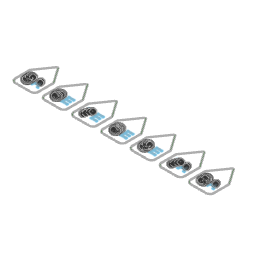
6-9 (Autodesk Fusion 360 design; units mm, degrees)
Autodesk Fusion 360 part; units mm, degrees
(part 1 of 2)
sketch "Sketch1" plane through (0, 0, 1) normal (0, 0, 1) x (-1, 0, 0)
  arc A0 (14.0709, -45.9158) -> (17.3475, -45.9158) centre (15.7092, -44.7687) ccw
  line L0 (17.3475, -45.9158) -> (31.3664, -25.8947)
  arc A1 (31.3664, -25.8947) -> (31.7281, -24.7475) centre (29.7281, -24.7475) ccw
  line L1 (31.7281, -24.7475) -> (31.7281, -6.3281)
  arc A2 (31.7281, -6.3281) -> (25.4, 0) centre (25.4, -6.3281) ccw
  line L2 (25.4, 0) -> (6.0183, 0)
  arc A3 (6.0183, 0) -> (0, -4.3724) centre (6.0183, -6.3281) ccw
  line L3 (0, -4.3724) -> (0, -25.19)
  arc A4 (0, -25.19) -> (0.3617, -26.3371) centre (2, -25.19) ccw
  line L4 (0.3617, -26.3371) -> (14.0709, -45.9158)
  arc A5 (-24.0291, -45.9158) -> (-20.7525, -45.9158) centre (-22.3908, -44.7687) ccw
  line L5 (-20.7525, -45.9158) -> (-6.7336, -25.8947)
  arc A6 (-6.7336, -25.8947) -> (-6.3719, -24.7475) centre (-8.3719, -24.7475) ccw
  line L6 (-6.3719, -24.7475) -> (-6.3719, -6.3281)
  arc A7 (-6.3719, -6.3281) -> (-12.7, 0) centre (-12.7, -6.3281) ccw
  line L7 (-12.7, 0) -> (-32.0817, 0)
  arc A8 (-32.0817, 0) -> (-38.1, -4.3724) centre (-32.0817, -6.3281) ccw
  line L8 (-38.1, -4.3724) -> (-38.1, -25.19)
  arc A9 (-38.1, -25.19) -> (-37.7383, -26.3371) centre (-36.1, -25.19) ccw
  line L9 (-37.7383, -26.3371) -> (-24.0291, -45.9158)
  arc A10 (-62.1291, -45.9158) -> (-58.8525, -45.9158) centre (-60.4908, -44.7687) ccw
  line L10 (-58.8525, -45.9158) -> (-44.8336, -25.8947)
  arc A11 (-44.8336, -25.8947) -> (-44.4719, -24.7475) centre (-46.4719, -24.7475) ccw
  line L11 (-44.4719, -24.7475) -> (-44.4719, -6.3281)
  arc A12 (-44.4719, -6.3281) -> (-50.8, 0) centre (-50.8, -6.3281) ccw
  line L12 (-50.8, 0) -> (-70.1817, 0)
  arc A13 (-70.1817, 0) -> (-76.2, -4.3724) centre (-70.1817, -6.3281) ccw
  line L13 (-76.2, -4.3724) -> (-76.2, -25.19)
  arc A14 (-76.2, -25.19) -> (-75.8383, -26.3371) centre (-74.2, -25.19) ccw
  line L14 (-75.8383, -26.3371) -> (-62.1291, -45.9158)
  arc A15 (-100.2291, -45.9158) -> (-96.9525, -45.9158) centre (-98.5908, -44.7687) ccw
  line L15 (-96.9525, -45.9158) -> (-82.9336, -25.8947)
  arc A16 (-82.9336, -25.8947) -> (-82.5719, -24.7475) centre (-84.5719, -24.7475) ccw
  line L16 (-82.5719, -24.7475) -> (-82.5719, -6.3281)
  arc A17 (-82.5719, -6.3281) -> (-88.9, 0) centre (-88.9, -6.3281) ccw
  line L17 (-88.9, 0) -> (-108.2817, 0)
  arc A18 (-108.2817, 0) -> (-114.3, -4.3724) centre (-108.2817, -6.3281) ccw
  line L18 (-114.3, -4.3724) -> (-114.3, -25.19)
  arc A19 (-114.3, -25.19) -> (-113.9383, -26.3371) centre (-112.3, -25.19) ccw
  line L19 (-113.9383, -26.3371) -> (-100.2291, -45.9158)
  arc A20 (-138.3291, -45.9158) -> (-135.0525, -45.9158) centre (-136.6908, -44.7687) ccw
  line L20 (-135.0525, -45.9158) -> (-121.0336, -25.8947)
  arc A21 (-121.0336, -25.8947) -> (-120.6719, -24.7475) centre (-122.6719, -24.7475) ccw
  line L21 (-120.6719, -24.7475) -> (-120.6719, -6.3281)
  arc A22 (-120.6719, -6.3281) -> (-127, 0) centre (-127, -6.3281) ccw
  line L22 (-127, 0) -> (-146.3817, 0)
  arc A23 (-146.3817, 0) -> (-152.4, -4.3724) centre (-146.3817, -6.3281) ccw
  line L23 (-152.4, -4.3724) -> (-152.4, -25.19)
  arc A24 (-152.4, -25.19) -> (-152.0383, -26.3371) centre (-150.4, -25.19) ccw
  line L24 (-152.0383, -26.3371) -> (-138.3291, -45.9158)
  arc A25 (-176.4291, -45.9158) -> (-173.1525, -45.9158) centre (-174.7908, -44.7687) ccw
  line L25 (-173.1525, -45.9158) -> (-159.1336, -25.8947)
  arc A26 (-159.1336, -25.8947) -> (-158.7719, -24.7475) centre (-160.7719, -24.7475) ccw
  line L26 (-158.7719, -24.7475) -> (-158.7719, -6.3281)
  arc A27 (-158.7719, -6.3281) -> (-165.1, 0) centre (-165.1, -6.3281) ccw
  line L27 (-165.1, 0) -> (-184.4817, 0)
  arc A28 (-184.4817, 0) -> (-190.5, -4.3724) centre (-184.4817, -6.3281) ccw
  line L28 (-190.5, -4.3724) -> (-190.5, -25.19)
  arc A29 (-190.5, -25.19) -> (-190.1383, -26.3371) centre (-188.5, -25.19) ccw
  line L29 (-190.1383, -26.3371) -> (-176.4291, -45.9158)
  arc A30 (-214.5291, -45.9158) -> (-211.2525, -45.9158) centre (-212.8908, -44.7687) ccw
  line L30 (-211.2525, -45.9158) -> (-197.2336, -25.8947)
  arc A31 (-197.2336, -25.8947) -> (-196.8719, -24.7475) centre (-198.8719, -24.7475) ccw
  line L31 (-196.8719, -24.7475) -> (-196.8719, -6.3281)
  arc A32 (-196.8719, -6.3281) -> (-203.2, 0) centre (-203.2, -6.3281) ccw
  line L32 (-203.2, 0) -> (-222.5817, 0)
  arc A33 (-222.5817, 0) -> (-228.6, -4.3724) centre (-222.5817, -6.3281) ccw
  line L33 (-228.6, -4.3724) -> (-228.6, -25.19)
  arc A34 (-228.6, -25.19) -> (-228.2383, -26.3371) centre (-226.6, -25.19) ccw
  line L34 (-228.2383, -26.3371) -> (-214.5291, -45.9158)
  line L35 (16.1187, -45.0555) -> (30.1377, -25.0343)
  arc A35 (30.1377, -25.0343) -> (30.2281, -24.7475) centre (29.7281, -24.7475) ccw
  line L36 (30.2281, -24.7475) -> (30.2281, -6.3281)
  arc A36 (30.2281, -6.3281) -> (25.4, -1.5) centre (25.4, -6.3281) ccw
  line L37 (25.4, -1.5) -> (6.0183, -1.5)
  arc A37 (6.0183, -1.5) -> (1.5, -4.6265) centre (6.0183, -6.3281) ccw
  line L38 (1.5, -4.6265) -> (1.5, -25.19)
  arc A38 (1.5, -25.19) -> (1.5904, -25.4768) centre (2, -25.19) ccw
  line L39 (1.5904, -25.4768) -> (15.2996, -45.0555)
  arc A39 (15.2996, -45.0555) -> (16.1187, -45.0555) centre (15.7092, -44.7687) ccw
  line L40 (-21.9813, -45.0555) -> (-7.9623, -25.0343)
  arc A40 (-7.9623, -25.0343) -> (-7.8719, -24.7475) centre (-8.3719, -24.7475) ccw
  line L41 (-7.8719, -24.7475) -> (-7.8719, -6.3281)
  arc A41 (-7.8719, -6.3281) -> (-12.7, -1.5) centre (-12.7, -6.3281) ccw
  line L42 (-12.7, -1.5) -> (-32.0817, -1.5)
  arc A42 (-32.0817, -1.5) -> (-36.6, -4.6265) centre (-32.0817, -6.3281) ccw
  line L43 (-36.6, -4.6265) -> (-36.6, -25.19)
  arc A43 (-36.6, -25.19) -> (-36.5096, -25.4768) centre (-36.1, -25.19) ccw
  line L44 (-36.5096, -25.4768) -> (-22.8004, -45.0555)
  arc A44 (-22.8004, -45.0555) -> (-21.9813, -45.0555) centre (-22.3908, -44.7687) ccw
  line L45 (-60.0813, -45.0555) -> (-46.0623, -25.0343)
  arc A45 (-46.0623, -25.0343) -> (-45.9719, -24.7475) centre (-46.4719, -24.7475) ccw
  line L46 (-45.9719, -24.7475) -> (-45.9719, -6.3281)
  arc A46 (-45.9719, -6.3281) -> (-50.8, -1.5) centre (-50.8, -6.3281) ccw
  line L47 (-50.8, -1.5) -> (-70.1817, -1.5)
  arc A47 (-70.1817, -1.5) -> (-74.7, -4.6265) centre (-70.1817, -6.3281) ccw
  line L48 (-74.7, -4.6265) -> (-74.7, -25.19)
  arc A48 (-74.7, -25.19) -> (-74.6096, -25.4768) centre (-74.2, -25.19) ccw
  line L49 (-74.6096, -25.4768) -> (-60.9004, -45.0555)
  arc A49 (-60.9004, -45.0555) -> (-60.0813, -45.0555) centre (-60.4908, -44.7687) ccw
  line L50 (-98.1813, -45.0555) -> (-84.1623, -25.0343)
  arc A50 (-84.1623, -25.0343) -> (-84.0719, -24.7475) centre (-84.5719, -24.7475) ccw
  line L51 (-84.0719, -24.7475) -> (-84.0719, -6.3281)
  arc A51 (-84.0719, -6.3281) -> (-88.9, -1.5) centre (-88.9, -6.3281) ccw
  line L52 (-88.9, -1.5) -> (-108.2817, -1.5)
  arc A52 (-108.2817, -1.5) -> (-112.8, -4.6265) centre (-108.2817, -6.3281) ccw
  line L53 (-112.8, -4.6265) -> (-112.8, -25.19)
  arc A53 (-112.8, -25.19) -> (-112.7096, -25.4768) centre (-112.3, -25.19) ccw
  line L54 (-112.7096, -25.4768) -> (-99.0004, -45.0555)
  arc A54 (-99.0004, -45.0555) -> (-98.1813, -45.0555) centre (-98.5908, -44.7687) ccw
  line L55 (-136.2813, -45.0555) -> (-122.2623, -25.0343)
  arc A55 (-122.2623, -25.0343) -> (-122.1719, -24.7475) centre (-122.6719, -24.7475) ccw
  line L56 (-122.1719, -24.7475) -> (-122.1719, -6.3281)
  arc A56 (-122.1719, -6.3281) -> (-127, -1.5) centre (-127, -6.3281) ccw
  line L57 (-127, -1.5) -> (-146.3817, -1.5)
  arc A57 (-146.3817, -1.5) -> (-150.9, -4.6265) centre (-146.3817, -6.3281) ccw
  line L58 (-150.9, -4.6265) -> (-150.9, -25.19)
  arc A58 (-150.9, -25.19) -> (-150.8096, -25.4768) centre (-150.4, -25.19) ccw
  line L59 (-150.8096, -25.4768) -> (-137.1004, -45.0555)
  arc A59 (-137.1004, -45.0555) -> (-136.2813, -45.0555) centre (-136.6908, -44.7687) ccw
  line L60 (-160.2719, -24.7475) -> (-160.2719, -6.3281)
  arc A60 (-160.2719, -6.3281) -> (-165.1, -1.5) centre (-165.1, -6.3281) ccw
  line L61 (-165.1, -1.5) -> (-184.4817, -1.5)
  arc A61 (-184.4817, -1.5) -> (-189, -4.6265) centre (-184.4817, -6.3281) ccw
  line L62 (-189, -4.6265) -> (-189, -25.19)
  arc A62 (-189, -25.19) -> (-188.9096, -25.4768) centre (-188.5, -25.19) ccw
  line L63 (-188.9096, -25.4768) -> (-175.2004, -45.0555)
  arc A63 (-175.2004, -45.0555) -> (-174.3813, -45.0555) centre (-174.7908, -44.7687) ccw
  line L64 (-174.3813, -45.0555) -> (-160.3623, -25.0343)
  arc A64 (-160.3623, -25.0343) -> (-160.2719, -24.7475) centre (-160.7719, -24.7475) ccw
  line L65 (-212.4813, -45.0555) -> (-198.4623, -25.0343)
  arc A65 (-198.4623, -25.0343) -> (-198.3719, -24.7475) centre (-198.8719, -24.7475) ccw
  line L66 (-198.3719, -24.7475) -> (-198.3719, -6.3281)
  arc A66 (-198.3719, -6.3281) -> (-203.2, -1.5) centre (-203.2, -6.3281) ccw
  line L67 (-203.2, -1.5) -> (-222.5817, -1.5)
  arc A67 (-222.5817, -1.5) -> (-227.1, -4.6265) centre (-222.5817, -6.3281) ccw
  line L68 (-227.1, -4.6265) -> (-227.1, -25.19)
  arc A68 (-227.1, -25.19) -> (-227.0096, -25.4768) centre (-226.6, -25.19) ccw
  line L69 (-227.0096, -25.4768) -> (-213.3004, -45.0555)
  arc A69 (-213.3004, -45.0555) -> (-212.4813, -45.0555) centre (-212.8908, -44.7687) ccw
  line L70 (-7.9796, -5.9789) -> (-36.2077, -5.9789) construction
  line L71 (-36.2077, -5.9789) -> (-36.2077, -24.6143) construction
  line L72 (-36.2077, -24.6143) -> (-7.9796, -24.6143) construction
  line L73 (-7.9796, -24.6143) -> (-7.9796, -5.9789) construction
  line L74 (-46.2203, -6.1121) -> (-74.4484, -6.1121) construction
  line L75 (-74.4484, -6.1121) -> (-74.4484, -24.7475) construction
  line L76 (-74.4484, -24.7475) -> (-46.2203, -24.7475) construction
  line L77 (-46.2203, -24.7475) -> (-46.2203, -6.1121) construction
  line L78 (-84.8121, -6.1121) -> (-113.0403, -6.1121) construction
  line L79 (-113.0403, -6.1121) -> (-113.0403, -24.7475) construction
  line L80 (-113.0403, -24.7475) -> (-84.8121, -24.7475) construction
  line L81 (-84.8121, -24.7475) -> (-84.8121, -6.1121) construction
  line L82 (29.7281, -6.1121) -> (1.5, -6.1121) construction
  line L83 (1.5, -6.1121) -> (1.5, -24.7475) construction
  line L84 (1.5, -24.7475) -> (29.7281, -24.7475) construction
  line L85 (29.7281, -24.7475) -> (29.7281, -6.1121) construction
  line L86 (-122.5602, -5.9501) -> (-150.7883, -5.9501) construction
  line L87 (-150.7883, -5.9501) -> (-150.7883, -24.5855) construction
  line L88 (-150.7883, -24.5855) -> (-122.5602, -24.5855) construction
  line L89 (-122.5602, -24.5855) -> (-122.5602, -5.9501) construction
  line L90 (-160.6323, -6.4361) -> (-188.8604, -6.4361) construction
  line L91 (-188.8604, -6.4361) -> (-188.8604, -25.0715) construction
  line L92 (-188.8604, -25.0715) -> (-160.6323, -25.0715) construction
  line L93 (-160.6323, -25.0715) -> (-160.6323, -6.4361) construction
  line L94 (-199.0284, -6.1121) -> (-227.2565, -6.1121) construction
  line L95 (-227.2565, -6.1121) -> (-227.2565, -24.7475) construction
  line L96 (-227.2565, -24.7475) -> (-199.0284, -24.7475) construction
  line L97 (-199.0284, -24.7475) -> (-199.0284, -6.1121) construction
  dimension "d1" = -1.5
  dimension "d2" = -1.5
  dimension "d3" = -1.5
  dimension "d4" = -1.5
  dimension "d5" = -1.5
  dimension "d6" = -1.5
  dimension "d7" = -1.5
sketch "sketch 2408" plane through (0, 0, 1) normal (0, 0, 1) x (-1, 0, 0)
  line L0 (11.1666, -17.4709) -> (12.2657, -14.5356)
  spline S0 degree 3 poles (10.6273, -19.3824) (10.698, -19.0609) (10.8404, -18.4133) (11.0574, -17.7866) (11.1666, -17.4709) knots 0 0 0 0 0.09864 0.198754 0.198754 0.198754 0.198754
  spline S1 degree 3 poles (9.9174, -17.3071) (10.0605, -17.6891) (10.3171, -18.374) (10.5322, -19.0731) (10.6273, -19.3824) knots 0 0 0 0 0.122331 0.219376 0.219376 0.219376 0.219376
  line L1 (8.8729, -14.5356) -> (9.9174, -17.3071)
  line L2 (12.2657, -14.5356) -> (8.8729, -14.5356)
  line L3 (13.747, -10.426) -> (15.1533, -10.426)
  line L4 (12.648, -13.457) -> (13.747, -10.426)
  line L5 (8.4633, -13.457) -> (12.648, -13.457)
  line L6 (7.296, -10.426) -> (8.4633, -13.457)
  line L7 (5.7874, -10.426) -> (7.296, -10.426)
  line L8 (9.8832, -20.4336) -> (5.7874, -10.426)
  line L9 (11.31, -20.4336) -> (9.8832, -20.4336)
  line L10 (15.1533, -10.426) -> (11.31, -20.4336)
  spline S2 degree 3 poles (24.3622, -10.9073) (24.5865, -11.1558) (25.0592, -11.6795) (25.1885, -12.3748) (25.2564, -12.7402) knots 0 0 0 0 0.098474 0.207515 0.207515 0.207515 0.207515
  spline S3 degree 3 poles (22.4439, -10.2554) (22.8109, -10.277) (23.5118, -10.3184) (24.0878, -10.7173) (24.3622, -10.9073) knots 0 0 0 0 0.107902 0.2061 0.2061 0.2061 0.2061
  spline S4 degree 3 poles (20.5155, -10.8493) (20.8056, -10.6761) (21.3995, -10.3215) (22.0905, -10.2777) (22.4439, -10.2554) knots 0 0 0 0 0.099829 0.204395 0.204395 0.204395 0.204395
  spline S5 degree 3 poles (19.2765, -12.5798) (19.4252, -12.2287) (19.7093, -11.5582) (20.2553, -11.0781) (20.5155, -10.8493) knots 0 0 0 0 0.112701 0.215277 0.215277 0.215277 0.215277
  spline S6 degree 3 poles (18.86, -15.6346) (18.8678, -15.0564) (18.8817, -14.0198) (19.1554, -13.0213) (19.2765, -12.5798) knots 0 0 0 0 0.172597 0.309411 0.309411 0.309411 0.309411
  spline S7 degree 3 poles (19.2799, -18.4505) (19.158, -18.0565) (18.875, -17.1412) (18.8655, -16.1813) (18.86, -15.6346) knots 0 0 0 0 0.123131 0.286024 0.286024 0.286024 0.286024
  spline S8 degree 3 poles (20.5086, -19.9489) (20.2536, -19.7512) (19.7303, -19.3457) (19.4325, -18.7538) (19.2799, -18.4505) knots 0 0 0 0 0.095539 0.195973 0.195973 0.195973 0.195973
  spline S9 degree 3 poles (22.2938, -20.4746) (21.9758, -20.453) (21.3418, -20.4098) (20.7858, -20.1023) (20.5086, -19.9489) knots 0 0 0 0 0.094357 0.188122 0.188122 0.188122 0.188122
  spline S10 degree 3 poles (24.5431, -19.5462) (24.2221, -19.817) (23.5718, -20.3656) (22.7234, -20.4379) (22.2938, -20.4746) knots 0 0 0 0 0.122772 0.248744 0.248744 0.248744 0.248744
  spline S11 degree 3 poles (25.4408, -17.0955) (25.4107, -17.5703) (25.3532, -18.4783) (24.8048, -19.2013) (24.5431, -19.5462) knots 0 0 0 0 0.139204 0.266205 0.266205 0.266205 0.266205
  spline S12 degree 3 poles (24.5806, -14.7199) (24.8313, -15.0547) (25.3575, -15.7574) (25.4121, -16.6357) (25.4408, -17.0955) knots 0 0 0 0 0.122761 0.257603 0.257603 0.257603 0.257603
  spline S13 degree 3 poles (22.4781, -13.8188) (22.8764, -13.8564) (23.6736, -13.9318) (24.2781, -14.4571) (24.5806, -14.7199) knots 0 0 0 0 0.116876 0.233928 0.233928 0.233928 0.233928
  spline S14 degree 3 poles (21.0957, -14.184) (21.3133, -14.0775) (21.7497, -13.8638) (22.2348, -13.8338) (22.4781, -13.8188) knots 0 0 0 0 0.071895 0.144237 0.144237 0.144237 0.144237
  spline S15 degree 3 poles (20.0888, -15.1363) (20.2245, -14.9489) (20.5002, -14.5683) (20.8952, -14.3134) (21.0957, -14.184) knots 0 0 0 0 0.068756 0.139669 0.139669 0.139669 0.139669
  spline S16 degree 3 poles (20.082, -14.8905) (20.0824, -14.9247) (20.0835, -15.0066) (20.0868, -15.0885) (20.0888, -15.1363) knots 0 0 0 0 0.010241 0.024586 0.024586 0.024586 0.024586
  spline S17 degree 3 poles (20.2663, -13.3887) (20.2125, -13.6358) (20.1049, -14.1307) (20.0896, -14.637) (20.082, -14.8905) knots 0 0 0 0 0.075682 0.151595 0.151595 0.151595 0.151595
  spline S18 degree 3 poles (20.7237, -12.218) (20.6339, -12.3853) (20.4347, -12.7569) (20.326, -13.1646) (20.2663, -13.3887) knots 0 0 0 0 0.056785 0.126065 0.126065 0.126065 0.126065
  spline S19 degree 3 poles (21.4234, -11.5251) (21.2873, -11.6193) (21.0132, -11.809) (20.8206, -12.081) (20.7237, -12.218) knots 0 0 0 0 0.049245 0.099152 0.099152 0.099152 0.099152
  spline S20 degree 3 poles (22.4166, -11.2657) (22.2362, -11.275) (21.8868, -11.293) (21.5744, -11.4495) (21.4234, -11.5251) knots 0 0 0 0 0.053555 0.103651 0.103651 0.103651 0.103651
  spline S21 degree 3 poles (23.502, -11.6411) (23.3466, -11.5317) (23.0216, -11.3029) (22.624, -11.2784) (22.4166, -11.2657) knots 0 0 0 0 0.055907 0.116877 0.116877 0.116877 0.116877
  spline S22 degree 3 poles (24.0755, -12.8494) (24.0232, -12.5997) (23.9287, -12.1489) (23.6337, -11.7978) (23.502, -11.6411) knots 0 0 0 0 0.075096 0.135587 0.135587 0.135587 0.135587
  line L11 (25.2564, -12.7402) -> (24.0755, -12.8494)
  spline S23 degree 3 poles (20.7749, -15.5015) (20.6148, -15.7311) (20.2695, -16.2266) (20.2408, -16.8321) (20.2253, -17.1569) knots 0 0 0 0 0.082313 0.177599 0.177599 0.177599 0.177599
  spline S24 degree 3 poles (22.1777, -14.9042) (21.9073, -14.9276) (21.374, -14.9739) (20.9727, -15.3273) (20.7749, -15.5015) knots 0 0 0 0 0.079158 0.156093 0.156093 0.156093 0.156093
  spline S25 degree 3 poles (23.601, -15.5015) (23.3968, -15.3273) (22.986, -14.977) (22.4481, -14.9285) (22.1777, -14.9042) knots 0 0 0 0 0.07847 0.157795 0.157795 0.157795 0.157795
  spline S26 degree 3 poles (24.1779, -17.0545) (24.1578, -16.7552) (24.1193, -16.179) (23.7692, -15.7214) (23.601, -15.5015) knots 0 0 0 0 0.087803 0.168983 0.168983 0.168983 0.168983
  spline S27 degree 3 poles (23.5703, -18.7884) (23.7474, -18.5415) (24.1184, -18.0243) (24.1575, -17.3874) (24.1779, -17.0545) knots 0 0 0 0 0.089298 0.18708 0.18708 0.18708 0.18708
  spline S28 degree 3 poles (22.1436, -19.4574) (22.4105, -19.4266) (22.9596, -19.3631) (23.363, -18.9835) (23.5703, -18.7884) knots 0 0 0 0 0.078431 0.161374 0.161374 0.161374 0.161374
  spline S29 degree 3 poles (20.7885, -18.8362) (20.9836, -19.0174) (21.3674, -19.3739) (21.8877, -19.4299) (22.1436, -19.4574) knots 0 0 0 0 0.077583 0.152676 0.152676 0.152676 0.152676
  spline S30 degree 3 poles (20.2253, -17.1569) (20.2422, -17.4837) (20.2738, -18.098) (20.6244, -18.6009) (20.7885, -18.8362) knots 0 0 0 0 0.095927 0.180303 0.180303 0.180303 0.180303
sketch "sketch 2641" plane through (0, 0, 1) normal (0, 0, 1) x (-1, 0, 0)
  spline S0 degree 3 poles (-127.9261, -10.7453) (-127.7018, -10.9938) (-127.2291, -11.5175) (-127.0998, -12.2128) (-127.0319, -12.5782) knots 0 0 0 0 0.098474 0.207515 0.207515 0.207515 0.207515
  spline S1 degree 3 poles (-129.8444, -10.0934) (-129.4774, -10.115) (-128.7765, -10.1564) (-128.2005, -10.5553) (-127.9261, -10.7453) knots 0 0 0 0 0.107902 0.2061 0.2061 0.2061 0.2061
  spline S2 degree 3 poles (-131.7728, -10.6873) (-131.4828, -10.5141) (-130.8888, -10.1595) (-130.1979, -10.1157) (-129.8444, -10.0934) knots 0 0 0 0 0.099829 0.204395 0.204395 0.204395 0.204395
  spline S3 degree 3 poles (-133.0118, -12.4178) (-132.8631, -12.0667) (-132.579, -11.3962) (-132.033, -10.916) (-131.7728, -10.6873) knots 0 0 0 0 0.112701 0.215277 0.215277 0.215277 0.215277
  spline S4 degree 3 poles (-133.4283, -15.4726) (-133.4205, -14.8944) (-133.4066, -13.8578) (-133.1329, -12.8593) (-133.0118, -12.4178) knots 0 0 0 0 0.172597 0.309411 0.309411 0.309411 0.309411
  spline S5 degree 3 poles (-133.0084, -18.2885) (-133.1303, -17.8945) (-133.4134, -16.9792) (-133.4229, -16.0193) (-133.4283, -15.4726) knots 0 0 0 0 0.123131 0.286024 0.286024 0.286024 0.286024
  spline S6 degree 3 poles (-131.7797, -19.7869) (-132.0347, -19.5892) (-132.558, -19.1837) (-132.8558, -18.5918) (-133.0084, -18.2885) knots 0 0 0 0 0.095539 0.195973 0.195973 0.195973 0.195973
  spline S7 degree 3 poles (-129.9946, -20.3126) (-130.3126, -20.291) (-130.9466, -20.2478) (-131.5025, -19.9402) (-131.7797, -19.7869) knots 0 0 0 0 0.094357 0.188122 0.188122 0.188122 0.188122
  spline S8 degree 3 poles (-127.7452, -19.3842) (-128.0662, -19.6549) (-128.7165, -20.2035) (-129.5649, -20.2759) (-129.9946, -20.3126) knots 0 0 0 0 0.122772 0.248744 0.248744 0.248744 0.248744
  spline S9 degree 3 poles (-126.8476, -16.9335) (-126.8776, -17.4083) (-126.9351, -18.3163) (-127.4836, -19.0393) (-127.7452, -19.3842) knots 0 0 0 0 0.139204 0.266205 0.266205 0.266205 0.266205
  spline S10 degree 3 poles (-127.7077, -14.5579) (-127.457, -14.8927) (-126.9308, -15.5954) (-126.8762, -16.4737) (-126.8476, -16.9335) knots 0 0 0 0 0.122761 0.257603 0.257603 0.257603 0.257603
  spline S11 degree 3 poles (-129.8102, -13.6568) (-129.4119, -13.6944) (-128.6147, -13.7698) (-128.0102, -14.295) (-127.7077, -14.5579) knots 0 0 0 0 0.116876 0.233928 0.233928 0.233928 0.233928
  spline S12 degree 3 poles (-131.1926, -14.022) (-130.975, -13.9155) (-130.5386, -13.7018) (-130.0535, -13.6718) (-129.8102, -13.6568) knots 0 0 0 0 0.071895 0.144237 0.144237 0.144237 0.144237
  spline S13 degree 3 poles (-132.1995, -14.9743) (-132.0638, -14.7869) (-131.7881, -14.4063) (-131.3931, -14.1514) (-131.1926, -14.022) knots 0 0 0 0 0.068756 0.139669 0.139669 0.139669 0.139669
  spline S14 degree 3 poles (-132.2063, -14.7285) (-132.2059, -14.7627) (-132.2049, -14.8446) (-132.2015, -14.9265) (-132.1995, -14.9743) knots 0 0 0 0 0.010241 0.024586 0.024586 0.024586 0.024586
  spline S15 degree 3 poles (-132.022, -13.2267) (-132.0758, -13.4738) (-132.1835, -13.9687) (-132.1987, -14.475) (-132.2063, -14.7285) knots 0 0 0 0 0.075682 0.151595 0.151595 0.151595 0.151595
  spline S16 degree 3 poles (-131.5646, -12.056) (-131.6544, -12.2233) (-131.8536, -12.5949) (-131.9623, -13.0026) (-132.022, -13.2267) knots 0 0 0 0 0.056785 0.126065 0.126065 0.126065 0.126065
  spline S17 degree 3 poles (-130.8649, -11.3631) (-131.001, -11.4573) (-131.2751, -11.6469) (-131.4677, -11.919) (-131.5646, -12.056) knots 0 0 0 0 0.049245 0.099152 0.099152 0.099152 0.099152
  spline S18 degree 3 poles (-129.8717, -11.1037) (-130.0522, -11.113) (-130.4015, -11.1309) (-130.7139, -11.2874) (-130.8649, -11.3631) knots 0 0 0 0 0.053555 0.103651 0.103651 0.103651 0.103651
  spline S19 degree 3 poles (-128.7863, -11.4791) (-128.9417, -11.3697) (-129.2667, -11.1409) (-129.6643, -11.1164) (-129.8717, -11.1037) knots 0 0 0 0 0.055907 0.116877 0.116877 0.116877 0.116877
  spline S20 degree 3 poles (-128.2128, -12.6874) (-128.2651, -12.4377) (-128.3596, -11.9869) (-128.6546, -11.6358) (-128.7863, -11.4791) knots 0 0 0 0 0.075096 0.135587 0.135587 0.135587 0.135587
  line L0 (-127.0319, -12.5782) -> (-128.2128, -12.6874)
  spline S21 degree 3 poles (-131.5134, -15.3395) (-131.6735, -15.5691) (-132.0188, -16.0646) (-132.0476, -16.6701) (-132.063, -16.9949) knots 0 0 0 0 0.082313 0.177599 0.177599 0.177599 0.177599
  spline S22 degree 3 poles (-130.1106, -14.7422) (-130.381, -14.7656) (-130.9143, -14.8118) (-131.3156, -15.1653) (-131.5134, -15.3395) knots 0 0 0 0 0.079158 0.156093 0.156093 0.156093 0.156093
  spline S23 degree 3 poles (-128.6873, -15.3395) (-128.8916, -15.1653) (-129.3023, -14.8149) (-129.8402, -14.7665) (-130.1106, -14.7422) knots 0 0 0 0 0.07847 0.157795 0.157795 0.157795 0.157795
  spline S24 degree 3 poles (-128.1104, -16.8925) (-128.1305, -16.5931) (-128.169, -16.017) (-128.5191, -15.5593) (-128.6873, -15.3395) knots 0 0 0 0 0.087803 0.168983 0.168983 0.168983 0.168983
  spline S25 degree 3 poles (-128.718, -18.6264) (-128.5409, -18.3795) (-128.1699, -17.8623) (-128.1308, -17.2254) (-128.1104, -16.8925) knots 0 0 0 0 0.089298 0.18708 0.18708 0.18708 0.18708
  spline S26 degree 3 poles (-130.1447, -19.2954) (-129.8778, -19.2646) (-129.3287, -19.2011) (-128.9253, -18.8215) (-128.718, -18.6264) knots 0 0 0 0 0.078431 0.161374 0.161374 0.161374 0.161374
  spline S27 degree 3 poles (-131.4998, -18.6742) (-131.3047, -18.8554) (-130.9209, -19.2119) (-130.4006, -19.2679) (-130.1447, -19.2954) knots 0 0 0 0 0.077583 0.152676 0.152676 0.152676 0.152676
  spline S28 degree 3 poles (-132.063, -16.9949) (-132.0461, -17.3217) (-132.0145, -17.936) (-131.6639, -18.4389) (-131.4998, -18.6742) knots 0 0 0 0 0.095927 0.180303 0.180303 0.180303 0.180303
  line L1 (-146.5009, -10.264) -> (-139.0328, -10.264)
  line L2 (-146.5009, -11.445) -> (-146.5009, -10.264)
  line L3 (-140.3571, -11.445) -> (-146.5009, -11.445)
  line L4 (-140.3571, -14.8514) -> (-140.3571, -11.445)
  line L5 (-145.8934, -14.8514) -> (-140.3571, -14.8514)
  line L6 (-145.8934, -16.0256) -> (-145.8934, -14.8514)
  line L7 (-140.3571, -16.0256) -> (-145.8934, -16.0256)
  line L8 (-140.3571, -19.0906) -> (-140.3571, -16.0256)
  line L9 (-146.2688, -19.0906) -> (-140.3571, -19.0906)
  line L10 (-146.2688, -20.2716) -> (-146.2688, -19.0906)
  line L11 (-139.0328, -20.2716) -> (-146.2688, -20.2716)
  line L12 (-139.0328, -10.264) -> (-139.0328, -20.2716)
sketch "sketch 2864" plane through (0, 0, 1) normal (0, 0, 1) x (-1, 0, 0)
  spline S0 degree 3 poles (-89.5876, -14.9554) (-89.7754, -15.1588) (-90.1656, -15.5814) (-90.7132, -15.7603) (-90.9972, -15.8531) knots 0 0 0 0 0.081642 0.16962 0.16962 0.16962 0.16962
  spline S1 degree 3 poles (-89.0927, -13.3204) (-89.1092, -13.6271) (-89.141, -14.2135) (-89.4433, -14.7157) (-89.5876, -14.9554) knots 0 0 0 0 0.090532 0.173151 0.173151 0.173151 0.173151
  spline S2 degree 3 poles (-90.0006, -11.1326) (-89.7358, -11.4453) (-89.2005, -12.0774) (-89.1289, -12.9032) (-89.0927, -13.3204) knots 0 0 0 0 0.119793 0.242148 0.242148 0.242148 0.242148
  spline S3 degree 3 poles (-92.3898, -10.2554) (-91.9274, -10.2849) (-91.042, -10.3416) (-90.3373, -10.8769) (-90.0006, -11.1326) knots 0 0 0 0 0.135584 0.259601 0.259601 0.259601 0.259601
  spline S4 degree 3 poles (-94.7791, -11.1292) (-94.4423, -10.8744) (-93.737, -10.341) (-92.8522, -10.2847) (-92.3898, -10.2554) knots 0 0 0 0 0.123881 0.259451 0.259451 0.259451 0.259451
  spline S5 degree 3 poles (-95.687, -13.2863) (-95.65, -12.8764) (-95.5763, -12.0606) (-95.0439, -11.4386) (-94.7791, -11.1292) knots 0 0 0 0 0.120259 0.239281 0.239281 0.239281 0.239281
  spline S6 degree 3 poles (-95.2058, -14.8837) (-95.3461, -14.6452) (-95.636, -14.1525) (-95.6697, -13.5811) (-95.687, -13.2863) knots 0 0 0 0 0.081781 0.16897 0.16897 0.16897 0.16897
  spline S7 degree 3 poles (-93.8029, -15.8531) (-94.0879, -15.7428) (-94.634, -15.5316) (-95.0208, -15.0933) (-95.2058, -14.8837) knots 0 0 0 0 0.090144 0.172753 0.172753 0.172753 0.172753
  spline S8 degree 3 poles (-94.9122, -16.6483) (-94.7679, -16.4839) (-94.4604, -16.1336) (-94.0308, -15.9503) (-93.8029, -15.8531) knots 0 0 0 0 0.064803 0.138045 0.138045 0.138045 0.138045
  spline S9 degree 3 poles (-95.2774, -17.86) (-95.2639, -17.6379) (-95.2374, -17.2048) (-95.0187, -16.8306) (-94.9122, -16.6483) knots 0 0 0 0 0.065745 0.128141 0.128141 0.128141 0.128141
  spline S10 degree 3 poles (-94.4787, -19.7134) (-94.7117, -19.4464) (-95.1763, -18.914) (-95.2438, -18.2107) (-95.2774, -17.86) knots 0 0 0 0 0.103491 0.206393 0.206393 0.206393 0.206393
  spline S11 degree 3 poles (-92.3694, -20.4746) (-92.7778, -20.4494) (-93.5574, -20.4013) (-94.1816, -19.9353) (-94.4787, -19.7134) knots 0 0 0 0 0.11979 0.228631 0.228631 0.228631 0.228631
  spline S12 degree 3 poles (-90.2805, -19.7305) (-90.574, -19.9474) (-91.1933, -20.4048) (-91.964, -20.4505) (-92.3694, -20.4746) knots 0 0 0 0 0.107154 0.226034 0.226034 0.226034 0.226034
  spline S13 degree 3 poles (-89.4954, -17.8942) (-89.5278, -18.2434) (-89.5923, -18.9399) (-90.0515, -19.4675) (-90.2805, -19.7305) knots 0 0 0 0 0.102418 0.204272 0.204272 0.204272 0.204272
  spline S14 degree 3 poles (-89.8641, -16.6518) (-89.7566, -16.8371) (-89.5339, -17.2211) (-89.5086, -17.6647) (-89.4954, -17.8942) knots 0 0 0 0 0.063352 0.131221 0.131221 0.131221 0.131221
  spline S15 degree 3 poles (-90.9972, -15.8531) (-90.7636, -15.9499) (-90.3251, -16.1318) (-90.0109, -16.4862) (-89.8641, -16.6518) knots 0 0 0 0 0.074722 0.140252 0.140252 0.140252 0.140252
  spline S16 degree 3 poles (-91.2157, -19.0137) (-91.0803, -18.857) (-90.8118, -18.5462) (-90.7715, -18.1377) (-90.7515, -17.9351) knots 0 0 0 0 0.060511 0.120019 0.120019 0.120019 0.120019
  spline S17 degree 3 poles (-92.383, -19.4643) (-92.1605, -19.4473) (-91.7256, -19.4142) (-91.383, -19.1451) (-91.2157, -19.0137) knots 0 0 0 0 0.065318 0.127663 0.127663 0.127663 0.127663
  spline S18 degree 3 poles (-93.5469, -19.0035) (-93.3797, -19.1379) (-93.0396, -19.4111) (-92.6043, -19.4464) (-92.383, -19.4643) knots 0 0 0 0 0.062836 0.127778 0.127778 0.127778 0.127778
  spline S19 degree 3 poles (-94.0145, -17.8669) (-93.9957, -18.0826) (-93.9583, -18.5104) (-93.6833, -18.84) (-93.5469, -19.0035) knots 0 0 0 0 0.063295 0.125565 0.125565 0.125565 0.125565
  spline S20 degree 3 poles (-93.5606, -16.7712) (-93.693, -16.9292) (-93.9591, -17.2467) (-93.996, -17.6595) (-94.0145, -17.8669) knots 0 0 0 0 0.060283 0.121167 0.121167 0.121167 0.121167
  spline S21 degree 3 poles (-92.3967, -16.3241) (-92.6202, -16.3404) (-93.0541, -16.3719) (-93.3952, -16.6408) (-93.5606, -16.7712) knots 0 0 0 0 0.065555 0.12726 0.12726 0.12726 0.12726
  spline S22 degree 3 poles (-91.2089, -16.7746) (-91.3768, -16.6433) (-91.7253, -16.3707) (-92.1676, -16.34) (-92.3967, -16.3241) knots 0 0 0 0 0.062488 0.129656 0.129656 0.129656 0.129656
  spline S23 degree 3 poles (-90.7515, -17.9351) (-90.7683, -17.7116) (-90.801, -17.2767) (-91.0755, -16.9388) (-91.2089, -16.7746) knots 0 0 0 0 0.065516 0.127427 0.127427 0.127427 0.127427
  spline S24 degree 3 poles (-90.9256, -14.7472) (-90.7593, -14.5417) (-90.421, -14.1234) (-90.3776, -13.5867) (-90.3556, -13.3136) knots 0 0 0 0 0.07739 0.157513 0.157513 0.157513 0.157513
  spline S25 degree 3 poles (-92.3625, -15.3206) (-92.0879, -15.2986) (-91.5491, -15.2556) (-91.1307, -14.9144) (-90.9256, -14.7472) knots 0 0 0 0 0.080558 0.158019 0.158019 0.158019 0.158019
  spline S26 degree 3 poles (-93.8405, -14.7404) (-93.6285, -14.9096) (-93.1961, -15.2547) (-92.644, -15.2984) (-92.3625, -15.3206) knots 0 0 0 0 0.079451 0.162055 0.162055 0.162055 0.162055
  spline S27 degree 3 poles (-94.431, -13.2727) (-94.4083, -13.5537) (-94.364, -14.105) (-94.0127, -14.5313) (-93.8405, -14.7404) knots 0 0 0 0 0.082398 0.161634 0.161634 0.161634 0.161634
  spline S28 degree 3 poles (-93.8575, -11.8323) (-94.0248, -12.0371) (-94.367, -12.4563) (-94.4093, -12.9965) (-94.431, -13.2727) knots 0 0 0 0 0.07739 0.158368 0.158368 0.158368 0.158368
  spline S29 degree 3 poles (-92.4035, -11.2657) (-92.6817, -11.2869) (-93.2248, -11.3282) (-93.6501, -11.667) (-93.8575, -11.8323) knots 0 0 0 0 0.08162 0.159297 0.159297 0.159297 0.159297
  spline S30 degree 3 poles (-91.3454, -11.5353) (-91.5126, -11.4567) (-91.848, -11.2989) (-92.218, -11.2768) (-92.4035, -11.2657) knots 0 0 0 0 0.054889 0.110085 0.110085 0.110085 0.110085
  spline S31 degree 3 poles (-90.6047, -12.2965) (-90.6983, -12.1417) (-90.8862, -11.8307) (-91.1919, -11.6341) (-91.3454, -11.5353) knots 0 0 0 0 0.053486 0.107467 0.107467 0.107467 0.107467
  spline S32 degree 3 poles (-90.3556, -13.3136) (-90.3664, -13.1388) (-90.3885, -12.7849) (-90.5321, -12.4606) (-90.6047, -12.2965) knots 0 0 0 0 0.052084 0.105466 0.105466 0.105466 0.105466
  line L0 (-108.7597, -10.426) -> (-101.2916, -10.426)
  line L1 (-108.7597, -11.607) -> (-108.7597, -10.426)
  line L2 (-102.6159, -11.607) -> (-108.7597, -11.607)
  line L3 (-102.6159, -15.0134) -> (-102.6159, -11.607)
  line L4 (-108.1522, -15.0134) -> (-102.6159, -15.0134)
  line L5 (-108.1522, -16.1876) -> (-108.1522, -15.0134)
  line L6 (-102.6159, -16.1876) -> (-108.1522, -16.1876)
  line L7 (-102.6159, -19.2526) -> (-102.6159, -16.1876)
  line L8 (-108.5276, -19.2526) -> (-102.6159, -19.2526)
  line L9 (-108.5276, -20.4336) -> (-108.5276, -19.2526)
  line L10 (-101.2916, -20.4336) -> (-108.5276, -20.4336)
  line L11 (-101.2916, -10.426) -> (-101.2916, -20.4336)
sketch "sketch 3108" plane through (0, 0, 1) normal (0, 0, 1) x (-1, 0, 0)
  line L0 (-215.0163, -10.426) -> (-213.61, -10.426)
  line L1 (-216.1153, -13.457) -> (-215.0163, -10.426)
  line L2 (-220.3, -13.457) -> (-216.1153, -13.457)
  line L3 (-221.4673, -10.426) -> (-220.3, -13.457)
  line L4 (-222.9759, -10.426) -> (-221.4673, -10.426)
  line L5 (-218.8801, -20.4336) -> (-222.9759, -10.426)
  line L6 (-217.4533, -20.4336) -> (-218.8801, -20.4336)
  line L7 (-213.61, -10.426) -> (-217.4533, -20.4336)
  line L8 (-217.5967, -17.4709) -> (-216.4976, -14.5356)
  spline S0 degree 3 poles (-218.136, -19.3824) (-218.0653, -19.0609) (-217.9229, -18.4133) (-217.706, -17.7866) (-217.5967, -17.4709) knots 0 0 0 0 0.09864 0.198754 0.198754 0.198754 0.198754
  spline S1 degree 3 poles (-218.8459, -17.3071) (-218.7028, -17.6891) (-218.4462, -18.374) (-218.2311, -19.0731) (-218.136, -19.3824) knots 0 0 0 0 0.122331 0.219376 0.219376 0.219376 0.219376
  line L9 (-219.8904, -14.5356) -> (-218.8459, -17.3071)
  line L10 (-216.4976, -14.5356) -> (-219.8904, -14.5356)
  spline S2 degree 3 poles (-203.8038, -14.9554) (-203.9916, -15.1588) (-204.3818, -15.5814) (-204.9294, -15.7603) (-205.2135, -15.8531) knots 0 0 0 0 0.081642 0.16962 0.16962 0.16962 0.16962
  spline S3 degree 3 poles (-203.3089, -13.3204) (-203.3255, -13.6271) (-203.3572, -14.2135) (-203.6595, -14.7157) (-203.8038, -14.9554) knots 0 0 0 0 0.090532 0.173151 0.173151 0.173151 0.173151
  spline S4 degree 3 poles (-204.2168, -11.1326) (-203.952, -11.4453) (-203.4167, -12.0774) (-203.3451, -12.9032) (-203.3089, -13.3204) knots 0 0 0 0 0.119793 0.242148 0.242148 0.242148 0.242148
  spline S5 degree 3 poles (-206.6061, -10.2554) (-206.1437, -10.2849) (-205.2583, -10.3416) (-204.5535, -10.8769) (-204.2168, -11.1326) knots 0 0 0 0 0.135584 0.259601 0.259601 0.259601 0.259601
  spline S6 degree 3 poles (-208.9953, -11.1292) (-208.6586, -10.8744) (-207.9532, -10.341) (-207.0684, -10.2847) (-206.6061, -10.2554) knots 0 0 0 0 0.123881 0.259451 0.259451 0.259451 0.259451
  spline S7 degree 3 poles (-209.9033, -13.2863) (-209.8662, -12.8764) (-209.7925, -12.0606) (-209.2602, -11.4386) (-208.9953, -11.1292) knots 0 0 0 0 0.120259 0.239281 0.239281 0.239281 0.239281
  spline S8 degree 3 poles (-209.422, -14.8837) (-209.5623, -14.6452) (-209.8523, -14.1525) (-209.8859, -13.5811) (-209.9033, -13.2863) knots 0 0 0 0 0.081781 0.16897 0.16897 0.16897 0.16897
  spline S9 degree 3 poles (-208.0192, -15.8531) (-208.3041, -15.7428) (-208.8502, -15.5316) (-209.237, -15.0933) (-209.422, -14.8837) knots 0 0 0 0 0.090144 0.172753 0.172753 0.172753 0.172753
  spline S10 degree 3 poles (-209.1285, -16.6483) (-208.9841, -16.4839) (-208.6766, -16.1336) (-208.2471, -15.9503) (-208.0192, -15.8531) knots 0 0 0 0 0.064803 0.138045 0.138045 0.138045 0.138045
  spline S11 degree 3 poles (-209.4937, -17.86) (-209.4801, -17.6379) (-209.4537, -17.2048) (-209.235, -16.8306) (-209.1285, -16.6483) knots 0 0 0 0 0.065744 0.128141 0.128141 0.128141 0.128141
  spline S12 degree 3 poles (-208.695, -19.7134) (-208.9279, -19.4464) (-209.3925, -18.914) (-209.46, -18.2107) (-209.4937, -17.86) knots 0 0 0 0 0.103491 0.206393 0.206393 0.206393 0.206393
  spline S13 degree 3 poles (-206.5856, -20.4746) (-206.994, -20.4494) (-207.7736, -20.4013) (-208.3978, -19.9353) (-208.695, -19.7134) knots 0 0 0 0 0.11979 0.228631 0.228631 0.228631 0.228631
  spline S14 degree 3 poles (-204.4967, -19.7305) (-204.7903, -19.9474) (-205.4095, -20.4048) (-206.1803, -20.4505) (-206.5856, -20.4746) knots 0 0 0 0 0.107154 0.226034 0.226034 0.226034 0.226034
  spline S15 degree 3 poles (-203.7117, -17.8942) (-203.744, -18.2434) (-203.8085, -18.9399) (-204.2677, -19.4675) (-204.4967, -19.7305) knots 0 0 0 0 0.102418 0.204272 0.204272 0.204272 0.204272
  spline S16 degree 3 poles (-204.0803, -16.6518) (-203.9728, -16.8371) (-203.7502, -17.2211) (-203.7248, -17.6647) (-203.7117, -17.8942) knots 0 0 0 0 0.063352 0.131221 0.131221 0.131221 0.131221
  spline S17 degree 3 poles (-205.2135, -15.8531) (-204.9799, -15.9499) (-204.5414, -16.1318) (-204.2271, -16.4862) (-204.0803, -16.6518) knots 0 0 0 0 0.074722 0.140252 0.140252 0.140252 0.140252
  spline S18 degree 3 poles (-205.1418, -14.7472) (-204.9756, -14.5417) (-204.6372, -14.1234) (-204.5939, -13.5867) (-204.5718, -13.3136) knots 0 0 0 0 0.07739 0.157513 0.157513 0.157513 0.157513
  spline S19 degree 3 poles (-206.5788, -15.3206) (-206.3041, -15.2986) (-205.7653, -15.2556) (-205.3469, -14.9144) (-205.1418, -14.7472) knots 0 0 0 0 0.080558 0.158019 0.158019 0.158019 0.158019
  spline S20 degree 3 poles (-208.0567, -14.7404) (-207.8447, -14.9096) (-207.4124, -15.2547) (-206.8602, -15.2984) (-206.5788, -15.3206) knots 0 0 0 0 0.079451 0.162055 0.162055 0.162055 0.162055
  spline S21 degree 3 poles (-208.6472, -13.2727) (-208.6246, -13.5537) (-208.5802, -14.105) (-208.2289, -14.5313) (-208.0567, -14.7404) knots 0 0 0 0 0.082398 0.161634 0.161634 0.161634 0.161634
  spline S22 degree 3 poles (-208.0738, -11.8323) (-208.241, -12.0371) (-208.5832, -12.4563) (-208.6255, -12.9965) (-208.6472, -13.2727) knots 0 0 0 0 0.07739 0.158368 0.158368 0.158368 0.158368
  spline S23 degree 3 poles (-206.6197, -11.2657) (-206.898, -11.2869) (-207.441, -11.3282) (-207.8664, -11.667) (-208.0738, -11.8323) knots 0 0 0 0 0.08162 0.159297 0.159297 0.159297 0.159297
  spline S24 degree 3 poles (-205.5616, -11.5353) (-205.7289, -11.4567) (-206.0642, -11.2989) (-206.4342, -11.2768) (-206.6197, -11.2657) knots 0 0 0 0 0.054889 0.110085 0.110085 0.110085 0.110085
  spline S25 degree 3 poles (-204.821, -12.2965) (-204.9145, -12.1417) (-205.1024, -11.8307) (-205.4081, -11.6341) (-205.5616, -11.5353) knots 0 0 0 0 0.053486 0.107467 0.107467 0.107467 0.107467
  spline S26 degree 3 poles (-204.5718, -13.3136) (-204.5827, -13.1388) (-204.6047, -12.7849) (-204.7483, -12.4606) (-204.821, -12.2965) knots 0 0 0 0 0.052084 0.105466 0.105466 0.105466 0.105466
  spline S27 degree 3 poles (-205.4319, -19.0137) (-205.2965, -18.857) (-205.028, -18.5462) (-204.9877, -18.1377) (-204.9677, -17.9351) knots 0 0 0 0 0.060511 0.120019 0.120019 0.120019 0.120019
  spline S28 degree 3 poles (-206.5993, -19.4643) (-206.3767, -19.4473) (-205.9418, -19.4142) (-205.5992, -19.1451) (-205.4319, -19.0137) knots 0 0 0 0 0.065318 0.127663 0.127663 0.127663 0.127663
  spline S29 degree 3 poles (-207.7632, -19.0035) (-207.5959, -19.1379) (-207.2558, -19.4111) (-206.8205, -19.4464) (-206.5993, -19.4643) knots 0 0 0 0 0.062836 0.127778 0.127778 0.127778 0.127778
  spline S30 degree 3 poles (-208.2308, -17.8669) (-208.2119, -18.0826) (-208.1746, -18.5104) (-207.8996, -18.84) (-207.7632, -19.0035) knots 0 0 0 0 0.063295 0.125565 0.125565 0.125565 0.125565
  spline S31 degree 3 poles (-207.7768, -16.7712) (-207.9092, -16.9292) (-208.1754, -17.2467) (-208.2122, -17.6595) (-208.2308, -17.8669) knots 0 0 0 0 0.060283 0.121167 0.121167 0.121167 0.121167
  spline S32 degree 3 poles (-206.6129, -16.3241) (-206.8364, -16.3404) (-207.2704, -16.3719) (-207.6114, -16.6408) (-207.7768, -16.7712) knots 0 0 0 0 0.065555 0.12726 0.12726 0.12726 0.12726
  spline S33 degree 3 poles (-205.4251, -16.7746) (-205.5931, -16.6433) (-205.9415, -16.3707) (-206.3838, -16.34) (-206.6129, -16.3241) knots 0 0 0 0 0.062488 0.129656 0.129656 0.129656 0.129656
  spline S34 degree 3 poles (-204.9677, -17.9351) (-204.9845, -17.7116) (-205.0172, -17.2767) (-205.2917, -16.9388) (-205.4251, -16.7746) knots 0 0 0 0 0.065516 0.127427 0.127427 0.127427 0.127427
sketch "sketch 3361" plane through (0, 0, 1) normal (0, 0, 1) x (-1, 0, 0)
  spline S0 degree 3 poles (-17.7657, -19.6792) (-17.9929, -19.4295) (-18.468, -18.9073) (-18.6009, -18.2124) (-18.6702, -17.8497) knots 0 0 0 0 0.099278 0.207652 0.207652 0.207652 0.207652
  spline S1 degree 3 poles (-15.8304, -20.3413) (-16.2, -20.319) (-16.9077, -20.2763) (-17.4883, -19.8722) (-17.7657, -19.6792) knots 0 0 0 0 0.108699 0.208095 0.208095 0.208095 0.208095
  spline S2 degree 3 poles (-13.3114, -19.1945) (-13.6552, -19.529) (-14.3565, -20.2113) (-15.3327, -20.2974) (-15.8304, -20.3413) knots 0 0 0 0 0.139428 0.284452 0.284452 0.284452 0.284452
  spline S3 degree 3 poles (-12.2397, -14.9757) (-12.2526, -15.8322) (-12.2753, -17.332) (-13.0004, -18.6354) (-13.3114, -19.1945) knots 0 0 0 0 0.25196 0.441222 0.441222 0.441222 0.441222
  spline S4 degree 3 poles (-13.209, -11.2519) (-12.9278, -11.7393) (-12.2677, -12.8836) (-12.2499, -14.2128) (-12.2397, -14.9757) knots 0 0 0 0 0.166317 0.390429 0.390429 0.390429 0.390429
  spline S5 degree 3 poles (-15.7143, -10.1221) (-15.2274, -10.1675) (-14.2623, -10.2574) (-13.558, -10.9224) (-13.209, -11.2519) knots 0 0 0 0 0.142263 0.281988 0.281988 0.281988 0.281988
  spline S6 degree 3 poles (-17.3254, -10.5522) (-17.0776, -10.4268) (-16.5712, -10.1704) (-16.004, -10.1384) (-15.7143, -10.1221) knots 0 0 0 0 0.082353 0.168359 0.168359 0.168359 0.168359
  spline S7 degree 3 poles (-18.4415, -11.7912) (-18.2963, -11.5391) (-18.0124, -11.0462) (-17.5508, -10.7143) (-17.3254, -10.5522) knots 0 0 0 0 0.086171 0.168473 0.168473 0.168473 0.168473
  spline S8 degree 3 poles (-18.8477, -13.5422) (-18.8315, -13.2351) (-18.7994, -12.6274) (-18.56, -12.068) (-18.4415, -11.7912) knots 0 0 0 0 0.091443 0.181004 0.181004 0.181004 0.181004
  spline S9 degree 3 poles (-17.9841, -15.8802) (-18.2359, -15.5482) (-18.7593, -14.8579) (-18.8175, -13.9917) (-18.8477, -13.5422) knots 0 0 0 0 0.122244 0.254152 0.254152 0.254152 0.254152
  spline S10 degree 3 poles (-15.8918, -16.7848) (-16.2869, -16.7463) (-17.081, -16.6691) (-17.6821, -16.1441) (-17.9841, -15.8802) knots 0 0 0 0 0.115972 0.233102 0.233102 0.233102 0.233102
  spline S11 degree 3 poles (-14.547, -16.4571) (-14.7627, -16.5527) (-15.1914, -16.7426) (-15.6593, -16.7708) (-15.8918, -16.7848) knots 0 0 0 0 0.07015 0.139413 0.139413 0.139413 0.139413
  spline S12 degree 3 poles (-13.4616, -15.4536) (-13.6143, -15.6626) (-13.9108, -16.0683) (-14.3393, -16.3301) (-14.547, -16.4571) knots 0 0 0 0 0.076807 0.149103 0.149103 0.149103 0.149103
  spline S13 degree 3 poles (-13.8097, -17.7678) (-13.7118, -17.4417) (-13.4855, -16.6883) (-13.4703, -15.9004) (-13.4616, -15.4536) knots 0 0 0 0 0.101702 0.234978 0.234978 0.234978 0.234978
  spline S14 degree 3 poles (-14.7245, -19.0034) (-14.5387, -18.8395) (-14.1463, -18.4934) (-13.9258, -18.0181) (-13.8097, -17.7678) knots 0 0 0 0 0.073492 0.155229 0.155229 0.155229 0.155229
  spline S15 degree 3 poles (-15.7553, -19.331) (-15.5669, -19.3183) (-15.1962, -19.2933) (-14.88, -19.0989) (-14.7245, -19.0034) knots 0 0 0 0 0.055729 0.109615 0.109615 0.109615 0.109615
  spline S16 degree 3 poles (-16.9841, -18.8054) (-16.808, -18.9587) (-16.455, -19.2661) (-15.9889, -19.3093) (-15.7553, -19.331) knots 0 0 0 0 0.068187 0.1367 0.1367 0.1367 0.1367
  spline S17 degree 3 poles (-17.4483, -17.7541) (-17.3963, -17.9688) (-17.3045, -18.3483) (-17.0811, -18.667) (-16.9841, -18.8054) knots 0 0 0 0 0.065524 0.115815 0.115815 0.115815 0.115815
  line L0 (-18.6702, -17.8497) -> (-17.4483, -17.7541)
  spline S18 degree 3 poles (-14.233, -15.102) (-14.0638, -14.8811) (-13.7105, -14.4196) (-13.6725, -13.8383) (-13.6527, -13.5354) knots 0 0 0 0 0.081605 0.170432 0.170432 0.170432 0.170432
  spline S19 degree 3 poles (-15.6461, -15.6993) (-15.379, -15.6745) (-14.8448, -15.6247) (-14.4369, -15.2762) (-14.233, -15.102) knots 0 0 0 0 0.078404 0.156803 0.156803 0.156803 0.156803
  spline S20 degree 3 poles (-17.0387, -15.102) (-16.8412, -15.2762) (-16.4427, -15.6278) (-15.9132, -15.6753) (-15.6461, -15.6993) knots 0 0 0 0 0.076867 0.155103 0.155103 0.155103 0.155103
  spline S21 degree 3 poles (-17.5916, -13.4671) (-17.5754, -13.7868) (-17.545, -14.3861) (-17.1997, -14.8743) (-17.0387, -15.102) knots 0 0 0 0 0.093779 0.175778 0.175778 0.175778 0.175778
  spline S22 degree 3 poles (-17.0318, -11.7605) (-17.1949, -11.9995) (-17.5449, -12.5124) (-17.5753, -13.1347) (-17.5916, -13.4671) knots 0 0 0 0 0.085138 0.182741 0.182741 0.182741 0.182741
  spline S23 degree 3 poles (-15.6939, -11.1324) (-15.9461, -11.1609) (-16.4622, -11.219) (-16.8392, -11.5773) (-17.0318, -11.7605) knots 0 0 0 0 0.074044 0.151461 0.151461 0.151461 0.151461
  spline S24 degree 3 poles (-14.6767, -11.4362) (-14.8385, -11.3476) (-15.1561, -11.1737) (-15.5169, -11.146) (-15.6939, -11.1324) knots 0 0 0 0 0.054639 0.107242 0.107242 0.107242 0.107242
  spline S25 degree 3 poles (-13.9224, -12.3202) (-14.0187, -12.14) (-14.2057, -11.7898) (-14.5229, -11.5517) (-14.6767, -11.4362) knots 0 0 0 0 0.060485 0.117471 0.117471 0.117471 0.117471
  spline S26 degree 3 poles (-13.6527, -13.5354) (-13.6641, -13.3258) (-13.6868, -12.9059) (-13.8437, -12.5157) (-13.9224, -12.3202) knots 0 0 0 0 0.062485 0.125225 0.125225 0.125225 0.125225
  line L1 (-31.9477, -10.2928) -> (-24.4795, -10.2928)
  line L2 (-31.9477, -11.4738) -> (-31.9477, -10.2928)
  line L3 (-25.8038, -11.4738) -> (-31.9477, -11.4738)
  line L4 (-25.8038, -14.8802) -> (-25.8038, -11.4738)
  line L5 (-31.3401, -14.8802) -> (-25.8038, -14.8802)
  line L6 (-31.3401, -16.0543) -> (-31.3401, -14.8802)
  line L7 (-25.8038, -16.0543) -> (-31.3401, -16.0543)
  line L8 (-25.8038, -19.1194) -> (-25.8038, -16.0543)
  line L9 (-31.7156, -19.1194) -> (-25.8038, -19.1194)
  line L10 (-31.7156, -20.3004) -> (-31.7156, -19.1194)
  line L11 (-24.4795, -20.3004) -> (-31.7156, -20.3004)
  line L12 (-24.4795, -10.2928) -> (-24.4795, -20.3004)
sketch "sketch 3572" plane through (0, 0, 1) normal (0, 0, 1) x (-1, 0, 0)
  line L0 (-179.1528, -17.795) -> (-178.0538, -14.8596)
  spline S0 degree 3 poles (-179.6921, -19.7064) (-179.6214, -19.3849) (-179.479, -18.7373) (-179.2621, -18.1106) (-179.1528, -17.795) knots 0 0 0 0 0.09864 0.198754 0.198754 0.198754 0.198754
  spline S1 degree 3 poles (-180.4021, -17.6311) (-180.2589, -18.0131) (-180.0023, -18.698) (-179.7872, -19.3971) (-179.6921, -19.7064) knots 0 0 0 0 0.122331 0.219376 0.219376 0.219376 0.219376
  line L1 (-181.4465, -14.8596) -> (-180.4021, -17.6311)
  line L2 (-178.0538, -14.8596) -> (-181.4465, -14.8596)
  line L3 (-176.5724, -10.75) -> (-175.1662, -10.75)
  line L4 (-177.6715, -13.781) -> (-176.5724, -10.75)
  line L5 (-181.8561, -13.781) -> (-177.6715, -13.781)
  line L6 (-183.0234, -10.75) -> (-181.8561, -13.781)
  line L7 (-184.5321, -10.75) -> (-183.0234, -10.75)
  line L8 (-180.4362, -20.7576) -> (-184.5321, -10.75)
  line L9 (-179.0095, -20.7576) -> (-180.4362, -20.7576)
  line L10 (-175.1662, -10.75) -> (-179.0095, -20.7576)
  line L11 (-169.862, -19.447) -> (-164.9606, -19.447)
  spline S2 degree 3 poles (-168.0973, -16.829) (-168.3688, -17.3154) (-168.8835, -18.2379) (-169.5479, -19.0589) (-169.862, -19.447) knots 0 0 0 0 0.166741 0.316231 0.316231 0.316231 0.316231
  spline S3 degree 3 poles (-166.8242, -13.6035) (-166.9888, -14.1571) (-167.3194, -15.2693) (-167.8373, -16.3076) (-168.0973, -16.829) knots 0 0 0 0 0.172915 0.347351 0.347351 0.347351 0.347351
  spline S4 degree 3 poles (-166.36, -10.75) (-166.3906, -11.1865) (-166.4582, -12.1513) (-166.6947, -13.0896) (-166.8242, -13.6035) knots 0 0 0 0 0.130996 0.289598 0.289598 0.289598 0.289598
  line L12 (-167.6229, -10.75) -> (-166.36, -10.75)
  spline S5 degree 3 poles (-168.0939, -13.5011) (-167.9816, -13.0645) (-167.7491, -12.1606) (-167.6659, -11.2308) (-167.6229, -10.75) knots 0 0 0 0 0.135003 0.27952 0.27952 0.27952 0.27952
  spline S6 degree 3 poles (-169.5446, -16.969) (-169.2503, -16.406) (-168.6678, -15.2914) (-168.2839, -14.0938) (-168.0939, -13.5011) knots 0 0 0 0 0.190168 0.376518 0.376518 0.376518 0.376518
  spline S7 degree 3 poles (-171.4389, -19.6722) (-171.1103, -19.2856) (-170.3949, -18.4439) (-169.8429, -17.4865) (-169.5446, -16.969) knots 0 0 0 0 0.151922 0.330698 0.330698 0.330698 0.330698
  line L13 (-171.4389, -20.6279) -> (-171.4389, -19.6722)
  line L14 (-164.9606, -20.6279) -> (-171.4389, -20.6279)
  line L15 (-164.9606, -19.447) -> (-164.9606, -20.6279)